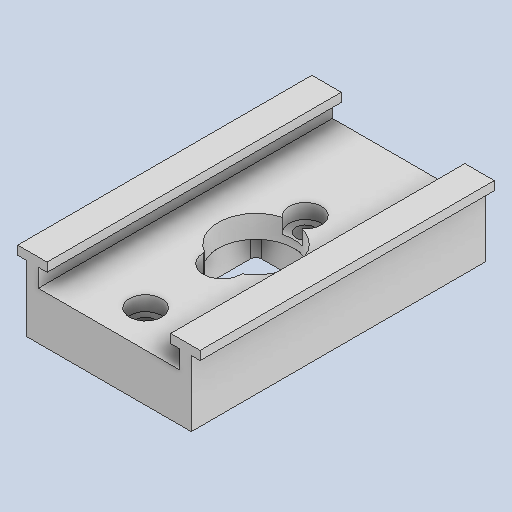
# Autodesk Inventor part: sg90 claw v2
Saved by Autodesk Inventor 2025 (Build 290162000, 162)
## iProperties
Created: 2025-05-11
Part Number: sg90 claw v2
Material: 一般
Document SubType Name: Modeling
Designer: gavin
Density: 1 g/cm^3
Appearance: 預設
Author: gavin
## iProperties of the stored document sg90 claw v2_3D 列印.ipt
Created: 2025-05-11
Part Number: sg90 claw v2_3D 列印
Material: 一般
Document SubType Name: Modeling
Designer: gavin
Density: 1 g/cm^3
Appearance: 預設
Author: gavin
Autodesk Inventor part; units mm, degrees
ref_plane "YZ Plane" through (0, 0, 0) normal (1, 0, 0) x (0, 1, 0)
sketch "草圖1" plane through (0, 0, 0) normal (0, 1, 0) x (-1, 0, 0)
  line L0 (-11.557, 4.8514) -> (-6.731, 4.8514) construction
  arc A0 (-11.557, 4.8514) -> (-12.192, 4.2164) centre (-11.557, 4.2164) ccw construction
  line L1 (-12.192, 4.2164) -> (-12.192, -0.635) construction
  arc A1 (-11.557, 0) -> (-12.192, -0.635) centre (-11.557, -0.635) ccw construction
  line L2 (-11.557, 0) -> (-0.635, 0) construction
  arc A2 (0, -0.635) -> (-0.635, 0) centre (-0.635, -0.635) ccw construction
  line L3 (0, 4.2164) -> (0, -0.635) construction
  arc A3 (0, 4.2164) -> (-0.635, 4.8514) centre (-0.635, 4.2164) ccw construction
  line L4 (-5.461, 4.8514) -> (-0.635, 4.8514) construction
  line L5 (-5.461, 4.0821) -> (-5.461, 4.8514) construction
  arc A4 (-6.731, 4.0821) -> (-5.461, 4.0821) centre (-6.096, 2.286) ccw construction
  line L6 (-6.731, 4.8514) -> (-6.731, 4.0821) construction
  line L7 (-12.192, -26.797) -> (-12.192, -21.9456) construction
  arc A5 (-12.192, -26.797) -> (-11.557, -27.432) centre (-11.557, -26.797) ccw construction
  line L8 (-11.557, -27.432) -> (-6.731, -27.432) construction
  line L9 (-6.731, -27.432) -> (-6.731, -26.6627) construction
  arc A6 (-5.461, -26.6627) -> (-6.731, -26.6627) centre (-6.096, -24.8666) ccw construction
  line L10 (-5.461, -26.6627) -> (-5.461, -27.432) construction
  line L11 (-5.461, -27.432) -> (-0.635, -27.432) construction
  arc A7 (-0.635, -27.432) -> (0, -26.797) centre (-0.635, -26.797) ccw construction
  line L12 (0, -26.797) -> (0, -21.9456) construction
  arc A8 (-0.635, -22.5806) -> (0, -21.9456) centre (-0.635, -21.9456) ccw construction
  line L13 (-11.557, -22.5806) -> (-0.635, -22.5806) construction
  arc A9 (-12.192, -21.9456) -> (-11.557, -22.5806) centre (-11.557, -21.9456) ccw construction
  line L14 (-20.096, 8.5154) -> (7.904, 8.5154)
  line L15 (7.904, 8.5154) -> (7.904, -41.4846)
  line L16 (7.904, -41.4846) -> (-20.096, -41.4846)
  line L17 (-20.096, -41.4846) -> (-20.096, 8.5154)
  line L18 (-20.096, 8.5154) -> (7.904, -41.4846) construction
  line L19 (7.904, 8.5154) -> (-20.096, -41.4846) construction
  arc A10 (-3.2258, -10.7188) -> (-8.9662, -10.7188) centre (-6.096, -10.7188) ccw construction
  line L20 (-8.9662, -10.7188) -> (-8.9662, -11.1066) construction
  arc A11 (-8.9662, -11.1066) -> (-3.2258, -11.1066) centre (-6.096, -16.4846) ccw construction
  line L21 (-3.2258, -11.1066) -> (-3.2258, -10.7188) construction
  arc A12 (-7.0699, -18.6923) -> (-7.0447, -18.7033) centre (-6.096, -16.4846) ccw construction
  spline S0 degree 3 poles (-7.0947, -18.3987) (-7.1625, -18.5159) (-7.1542, -18.6137) (-7.0699, -18.6923) knots 0.499854 0.499854 0.499854 0.499854 0.500096 0.500096 0.500096 0.500096 construction
  arc A13 (-7.336, -18.252) -> (-7.0947, -18.3987) centre (-6.096, -16.4846) ccw construction
  spline S1 degree 3 poles (-7.6081, -18.365) (-7.4996, -18.4037) (-7.4089, -18.3661) (-7.336, -18.252) knots 0.499904 0.499904 0.499904 0.499904 0.500146 0.500146 0.500146 0.500146 construction
  arc A14 (-7.6294, -18.3477) -> (-7.6081, -18.365) centre (-6.096, -16.4846) ccw construction
  spline S2 degree 3 poles (-7.5741, -18.0583) (-7.671, -18.1528) (-7.6894, -18.2493) (-7.6294, -18.3477) knots 0.499854 0.499854 0.499854 0.499854 0.500096 0.500096 0.500096 0.500096 construction
  arc A15 (-7.7669, -17.8519) -> (-7.5741, -18.0583) centre (-6.096, -16.4846) ccw construction
  spline S3 degree 3 poles (-8.0594, -17.8873) (-7.9653, -17.9539) (-7.8678, -17.9421) (-7.7669, -17.8519) knots 0.499904 0.499904 0.499904 0.499904 0.500146 0.500146 0.500146 0.500146 construction
  arc A16 (-8.0752, -17.8649) -> (-8.0594, -17.8873) centre (-6.096, -16.4846) ccw construction
  spline S4 degree 3 poles (-7.9439, -17.6011) (-8.0627, -17.666) (-8.1064, -17.7539) (-8.0752, -17.8649) knots 0.499854 0.499854 0.499854 0.499854 0.500096 0.500096 0.500096 0.500096 construction
  arc A17 (-8.0738, -17.3504) -> (-7.9439, -17.6011) centre (-6.096, -16.4846) ccw construction
  spline S5 degree 3 poles (-8.365, -17.3056) (-8.2924, -17.3951) (-8.1953, -17.41) (-8.0738, -17.3504) knots 0.499904 0.499904 0.499904 0.499904 0.500146 0.500146 0.500146 0.500146 construction
  arc A18 (-8.3742, -17.2797) -> (-8.365, -17.3056) centre (-6.096, -16.4846) ccw construction
  spline S6 degree 3 poles (-8.1766, -17.0612) (-8.3085, -17.0916) (-8.3744, -17.1644) (-8.3742, -17.2797) knots 0.499854 0.499854 0.499854 0.499854 0.500096 0.500096 0.500096 0.500096 construction
  arc A19 (-8.234, -16.7847) -> (-8.1766, -17.0612) centre (-6.096, -16.4846) ccw construction
  spline S7 degree 3 poles (-8.5024, -16.663) (-8.4566, -16.7687) (-8.3671, -16.8093) (-8.234, -16.7847) knots 0.499904 0.499904 0.499904 0.499904 0.500146 0.500146 0.500146 0.500146 construction
  arc A20 (-8.5043, -16.6356) -> (-8.5024, -16.663) centre (-6.096, -16.4846) ccw construction
  spline S8 degree 3 poles (-8.255, -16.4785) (-8.3902, -16.4722) (-8.4733, -16.5245) (-8.5043, -16.6356) knots 0.499854 0.499854 0.499854 0.499854 0.500096 0.500096 0.500096 0.500096 construction
  arc A21 (-8.2357, -16.1967) -> (-8.255, -16.4785) centre (-6.096, -16.4846) ccw construction
  spline S9 degree 3 poles (-8.4613, -16.0071) (-8.4457, -16.1213) (-8.3705, -16.1845) (-8.2357, -16.1967) knots 0.499904 0.499904 0.499904 0.499904 0.500146 0.500146 0.500146 0.500146 construction
  arc A22 (-8.4557, -15.9802) -> (-8.4613, -16.0071) centre (-6.096, -16.4846) ccw construction
  spline S10 degree 3 poles (-8.1733, -15.8962) (-8.3018, -15.8537) (-8.3959, -15.8817) (-8.4557, -15.9802) knots 0.499854 0.499854 0.499854 0.499854 0.500096 0.500096 0.500096 0.500096 construction
  arc A23 (-8.0787, -15.6301) -> (-8.1733, -15.8962) centre (-6.096, -16.4846) ccw construction
  spline S11 degree 3 poles (-8.2448, -15.3867) (-8.2606, -15.5008) (-8.2052, -15.582) (-8.0787, -15.6301) knots 0.499904 0.499904 0.499904 0.499904 0.500146 0.500146 0.500146 0.500146 construction
  arc A24 (-8.2321, -15.3623) -> (-8.2448, -15.3867) centre (-6.096, -16.4846) ccw construction
  spline S12 degree 3 poles (-7.9375, -15.3576) (-8.0497, -15.282) (-8.148, -15.2835) (-8.2321, -15.3623) knots 0.499854 0.499854 0.499854 0.499854 0.500096 0.500096 0.500096 0.500096 construction
  arc A25 (-7.7746, -15.1269) -> (-7.9375, -15.3576) centre (-6.096, -16.4846) ccw construction
  spline S13 degree 3 poles (-7.8689, -14.8477) (-7.9149, -14.9533) (-7.8835, -15.0464) (-7.7746, -15.1269) knots 0.499904 0.499904 0.499904 0.499904 0.500146 0.500146 0.500146 0.500146 construction
  arc A26 (-7.8501, -14.8276) -> (-7.8689, -14.8477) centre (-6.096, -16.4846) ccw construction
  spline S14 degree 3 poles (-7.5651, -14.9025) (-7.6528, -14.7994) (-7.7478, -14.7745) (-7.8501, -14.8276) knots 0.499854 0.499854 0.499854 0.499854 0.500096 0.500096 0.500096 0.500096 construction
  arc A27 (-7.3461, -14.7243) -> (-7.5651, -14.9025) centre (-6.096, -16.4846) ccw construction
  spline S15 degree 3 poles (-7.3615, -14.4301) (-7.4343, -14.5194) (-7.4292, -14.6175) (-7.3461, -14.7243) knots 0.499904 0.499904 0.499904 0.499904 0.500146 0.500146 0.500146 0.500146 construction
  arc A28 (-7.338, -14.4158) -> (-7.3615, -14.4301) centre (-6.096, -16.4846) ccw construction
  spline S16 degree 3 poles (-7.0838, -14.5648) (-7.1404, -14.4419) (-7.2252, -14.3922) (-7.338, -14.4158) knots 0.499854 0.499854 0.499854 0.499854 0.500096 0.500096 0.500096 0.500096 construction
  arc A29 (-6.8248, -14.4523) -> (-7.0838, -14.5648) centre (-6.096, -16.4846) ccw construction
  spline S17 degree 3 poles (-6.7602, -14.1648) (-6.8545, -14.2312) (-6.876, -14.327) (-6.8248, -14.4523) knots 0.499904 0.499904 0.499904 0.499904 0.500146 0.500146 0.500146 0.500146 construction
  arc A30 (-6.7338, -14.1574) -> (-6.7602, -14.1648) centre (-6.096, -16.4846) ccw construction
  spline S18 degree 3 poles (-6.5292, -14.3695) (-6.5506, -14.2359) (-6.6188, -14.1652) (-6.7338, -14.1574) knots 0.499854 0.499854 0.499854 0.499854 0.500096 0.500096 0.500096 0.500096 construction
  arc A31 (-6.2495, -14.3311) -> (-6.5292, -14.3695) centre (-6.096, -16.4846) ccw construction
  spline S19 degree 3 poles (-6.1097, -14.0716) (-6.2184, -14.1101) (-6.265, -14.1966) (-6.2495, -14.3311) knots 0.499904 0.499904 0.499904 0.499904 0.500146 0.500146 0.500146 0.500146 construction
  arc A32 (-6.0823, -14.0716) -> (-6.1097, -14.0716) centre (-6.096, -16.4846) ccw construction
  spline S20 degree 3 poles (-5.9425, -14.3311) (-5.927, -14.1966) (-5.9736, -14.1101) (-6.0823, -14.0716) knots 0.499854 0.499854 0.499854 0.499854 0.500096 0.500096 0.500096 0.500096 construction
  arc A33 (-5.6628, -14.3695) -> (-5.9425, -14.3311) centre (-6.096, -16.4846) ccw construction
  spline S21 degree 3 poles (-5.4582, -14.1574) (-5.5732, -14.1652) (-5.6414, -14.2359) (-5.6628, -14.3695) knots 0.499904 0.499904 0.499904 0.499904 0.500146 0.500146 0.500146 0.500146 construction
  arc A34 (-5.4318, -14.1648) -> (-5.4582, -14.1574) centre (-6.096, -16.4846) ccw construction
  spline S22 degree 3 poles (-5.3672, -14.4523) (-5.316, -14.327) (-5.3375, -14.2312) (-5.4318, -14.1648) knots 0.499854 0.499854 0.499854 0.499854 0.500096 0.500096 0.500096 0.500096 construction
  arc A35 (-5.1082, -14.5648) -> (-5.3672, -14.4523) centre (-6.096, -16.4846) ccw construction
  spline S23 degree 3 poles (-4.854, -14.4158) (-4.9668, -14.3922) (-5.0516, -14.4419) (-5.1082, -14.5648) knots 0.499904 0.499904 0.499904 0.499904 0.500146 0.500146 0.500146 0.500146 construction
  arc A36 (-4.8305, -14.4301) -> (-4.854, -14.4158) centre (-6.096, -16.4846) ccw construction
  spline S24 degree 3 poles (-4.8459, -14.7243) (-4.7628, -14.6175) (-4.7577, -14.5194) (-4.8305, -14.4301) knots 0.499854 0.499854 0.499854 0.499854 0.500096 0.500096 0.500096 0.500096 construction
  arc A37 (-4.6269, -14.9025) -> (-4.8459, -14.7243) centre (-6.096, -16.4846) ccw construction
  spline S25 degree 3 poles (-4.3419, -14.8276) (-4.4442, -14.7745) (-4.5392, -14.7994) (-4.6269, -14.9025) knots 0.499904 0.499904 0.499904 0.499904 0.500146 0.500146 0.500146 0.500146 construction
  arc A38 (-4.3231, -14.8477) -> (-4.3419, -14.8276) centre (-6.096, -16.4846) ccw construction
  spline S26 degree 3 poles (-4.4174, -15.1269) (-4.3085, -15.0464) (-4.2771, -14.9533) (-4.3231, -14.8477) knots 0.499854 0.499854 0.499854 0.499854 0.500096 0.500096 0.500096 0.500096 construction
  arc A39 (-4.2545, -15.3576) -> (-4.4174, -15.1269) centre (-6.096, -16.4846) ccw construction
  spline S27 degree 3 poles (-3.9599, -15.3623) (-4.044, -15.2835) (-4.1423, -15.282) (-4.2545, -15.3576) knots 0.499904 0.499904 0.499904 0.499904 0.500146 0.500146 0.500146 0.500146 construction
  arc A40 (-3.9472, -15.3867) -> (-3.9599, -15.3623) centre (-6.096, -16.4846) ccw construction
  spline S28 degree 3 poles (-4.1133, -15.6301) (-3.9868, -15.582) (-3.9314, -15.5008) (-3.9472, -15.3867) knots 0.499854 0.499854 0.499854 0.499854 0.500096 0.500096 0.500096 0.500096 construction
  arc A41 (-4.0187, -15.8962) -> (-4.1133, -15.6301) centre (-6.096, -16.4846) ccw construction
  spline S29 degree 3 poles (-3.7363, -15.9802) (-3.7961, -15.8817) (-3.8902, -15.8537) (-4.0187, -15.8962) knots 0.499904 0.499904 0.499904 0.499904 0.500146 0.500146 0.500146 0.500146 construction
  arc A42 (-3.7307, -16.0071) -> (-3.7363, -15.9802) centre (-6.096, -16.4846) ccw construction
  spline S30 degree 3 poles (-3.9563, -16.1967) (-3.8215, -16.1845) (-3.7463, -16.1213) (-3.7307, -16.0071) knots 0.499854 0.499854 0.499854 0.499854 0.500096 0.500096 0.500096 0.500096 construction
  arc A43 (-3.937, -16.4785) -> (-3.9563, -16.1967) centre (-6.096, -16.4846) ccw construction
  spline S31 degree 3 poles (-3.6877, -16.6356) (-3.7187, -16.5245) (-3.8018, -16.4722) (-3.937, -16.4785) knots 0.499904 0.499904 0.499904 0.499904 0.500146 0.500146 0.500146 0.500146 construction
  arc A44 (-3.6896, -16.663) -> (-3.6877, -16.6356) centre (-6.096, -16.4846) ccw construction
  spline S32 degree 3 poles (-3.958, -16.7847) (-3.8249, -16.8093) (-3.7354, -16.7687) (-3.6896, -16.663) knots 0.499854 0.499854 0.499854 0.499854 0.500096 0.500096 0.500096 0.500096 construction
  arc A45 (-4.0154, -17.0612) -> (-3.958, -16.7847) centre (-6.096, -16.4846) ccw construction
  spline S33 degree 3 poles (-3.8178, -17.2797) (-3.8176, -17.1644) (-3.8835, -17.0916) (-4.0154, -17.0612) knots 0.499904 0.499904 0.499904 0.499904 0.500146 0.500146 0.500146 0.500146 construction
  arc A46 (-3.827, -17.3056) -> (-3.8178, -17.2797) centre (-6.096, -16.4846) ccw construction
  spline S34 degree 3 poles (-4.1182, -17.3504) (-3.9967, -17.41) (-3.8996, -17.3951) (-3.827, -17.3056) knots 0.499854 0.499854 0.499854 0.499854 0.500096 0.500096 0.500096 0.500096 construction
  arc A47 (-4.2481, -17.6011) -> (-4.1182, -17.3504) centre (-6.096, -16.4846) ccw construction
  spline S35 degree 3 poles (-4.1168, -17.8649) (-4.0856, -17.7539) (-4.1293, -17.666) (-4.2481, -17.6011) knots 0.499904 0.499904 0.499904 0.499904 0.500146 0.500146 0.500146 0.500146 construction
  arc A48 (-4.1326, -17.8873) -> (-4.1168, -17.8649) centre (-6.096, -16.4846) ccw construction
  spline S36 degree 3 poles (-4.4251, -17.8519) (-4.3242, -17.9421) (-4.2267, -17.9539) (-4.1326, -17.8873) knots 0.499854 0.499854 0.499854 0.499854 0.500096 0.500096 0.500096 0.500096 construction
  arc A49 (-4.6179, -18.0583) -> (-4.4251, -17.8519) centre (-6.096, -16.4846) ccw construction
  spline S37 degree 3 poles (-4.5626, -18.3477) (-4.5026, -18.2493) (-4.521, -18.1528) (-4.6179, -18.0583) knots 0.499904 0.499904 0.499904 0.499904 0.500146 0.500146 0.500146 0.500146 construction
  arc A50 (-4.5839, -18.365) -> (-4.5626, -18.3477) centre (-6.096, -16.4846) ccw construction
  spline S38 degree 3 poles (-4.856, -18.252) (-4.7831, -18.3661) (-4.6924, -18.4037) (-4.5839, -18.365) knots 0.499854 0.499854 0.499854 0.499854 0.500096 0.500096 0.500096 0.500096 construction
  arc A51 (-5.0973, -18.3987) -> (-4.856, -18.252) centre (-6.096, -16.4846) ccw construction
  spline S39 degree 3 poles (-5.1221, -18.6923) (-5.0378, -18.6137) (-5.0295, -18.5159) (-5.0973, -18.3987) knots 0.499904 0.499904 0.499904 0.499904 0.500146 0.500146 0.500146 0.500146 construction
  arc A52 (-5.1473, -18.7033) -> (-5.1221, -18.6923) centre (-6.096, -16.4846) ccw construction
  spline S40 degree 3 poles (-5.3788, -18.521) (-5.3394, -18.6505) (-5.2623, -18.7113) (-5.1473, -18.7033) knots 0.499854 0.499854 0.499854 0.499854 0.500096 0.500096 0.500096 0.500096 construction
  arc A53 (-5.6507, -18.5972) -> (-5.3788, -18.521) centre (-6.096, -16.4846) ccw construction
  spline S41 degree 3 poles (-5.7538, -18.8732) (-5.6514, -18.8203) (-5.6171, -18.7283) (-5.6507, -18.5972) knots 0.499904 0.499904 0.499904 0.499904 0.500146 0.500146 0.500146 0.500146 construction
  arc A54 (-5.781, -18.877) -> (-5.7538, -18.8732) centre (-6.096, -16.4846) ccw construction
  spline S42 degree 3 poles (-5.9548, -18.639) (-5.9518, -18.7743) (-5.8939, -18.8536) (-5.781, -18.877) knots 0.499854 0.499854 0.499854 0.499854 0.500096 0.500096 0.500096 0.500096 construction
  arc A55 (-6.2372, -18.639) -> (-5.9548, -18.639) centre (-6.096, -16.4846) ccw construction
  spline S43 degree 3 poles (-6.411, -18.877) (-6.2981, -18.8536) (-6.2402, -18.7743) (-6.2372, -18.639) knots 0.499904 0.499904 0.499904 0.499904 0.500146 0.500146 0.500146 0.500146 construction
  arc A56 (-6.4382, -18.8732) -> (-6.411, -18.877) centre (-6.096, -16.4846) ccw construction
  spline S44 degree 3 poles (-6.5413, -18.5972) (-6.5749, -18.7283) (-6.5406, -18.8203) (-6.4382, -18.8732) knots 0.499854 0.499854 0.499854 0.499854 0.500096 0.500096 0.500096 0.500096 construction
  arc A57 (-6.8132, -18.521) -> (-6.5413, -18.5972) centre (-6.096, -16.4846) ccw construction
  spline S45 degree 3 poles (-7.0447, -18.7033) (-6.9297, -18.7113) (-6.8526, -18.6505) (-6.8132, -18.521) knots 0.499904 0.499904 0.499904 0.499904 0.500146 0.500146 0.500146 0.500146 construction
  line L22 (0, -16.4846) -> (0, -0.635) construction
  arc A58 (0, -0.635) -> (-0.635, 0) centre (-0.635, -0.635) ccw construction
  line L23 (-0.635, 0) -> (-11.557, 0) construction
  arc A59 (-11.557, 0) -> (-12.192, -0.635) centre (-11.557, -0.635) ccw construction
  line L24 (-12.192, -0.635) -> (-12.192, -16.4846) construction
  arc A60 (-8.9662, -11.1066) -> (-12.192, -16.4846) centre (-6.096, -16.4846) ccw construction
  line L25 (-8.9662, -10.7188) -> (-8.9662, -11.1066) construction
  arc A61 (-3.2258, -10.7188) -> (-8.9662, -10.7188) centre (-6.096, -10.7188) ccw construction
  line L26 (-3.2258, -11.1066) -> (-3.2258, -10.7188) construction
  arc A62 (0, -16.4846) -> (-3.2258, -11.1066) centre (-6.096, -16.4846) ccw construction
  line L27 (-6.096, -22.5806) -> (-0.635, -22.5806) construction
  arc A63 (-0.635, -22.5806) -> (0, -21.9456) centre (-0.635, -21.9456) ccw construction
  line L28 (0, -21.9456) -> (0, -16.4846) construction
  arc A64 (-6.096, -22.5806) -> (0, -16.4846) centre (-6.096, -16.4846) ccw construction
  line L29 (-12.192, -16.4846) -> (-12.192, -21.9456) construction
  arc A65 (-12.192, -21.9456) -> (-11.557, -22.5806) centre (-11.557, -21.9456) ccw construction
  line L30 (-11.557, -22.5806) -> (-6.096, -22.5806) construction
  arc A66 (-12.192, -16.4846) -> (-6.096, -22.5806) centre (-6.096, -16.4846) ccw construction
  line L31 (0.3, -0.635) -> (0.3, -16.4846)
  line L32 (0.3, -16.4846) -> (0.3, -21.9456)
  arc A67 (-0.635, -22.8806) -> (0.3, -21.9456) centre (-0.635, -21.9456) ccw
  line L33 (-0.635, -22.8806) -> (-6.096, -22.8806)
  line L34 (-6.096, -22.8806) -> (-11.557, -22.8806)
  arc A68 (-12.492, -21.9456) -> (-11.557, -22.8806) centre (-11.557, -21.9456) ccw
  line L35 (-12.492, -21.9456) -> (-12.492, -16.4846)
  line L36 (-12.492, -16.4846) -> (-12.492, -0.635)
  arc A69 (-11.557, 0.3) -> (-12.492, -0.635) centre (-11.557, -0.635) ccw
  line L37 (-11.557, 0.3) -> (-0.635, 0.3)
  arc A70 (0.3, -0.635) -> (-0.635, 0.3) centre (-0.635, -0.635) ccw
  circle A71 centre (-6.096, 2.286) radius 1.6
  circle A72 centre (-6.096, -24.8666) radius 1.6
  point P0 (0, 0)
  dimension "d0" = 28
  dimension "d1" = 50
  dimension "d2" = 0.3
  dimension "d3" = 3.2
  dimension "d4" = 3.2
  constraints: 26 end point, 8 point on circle, 6 centre point, 3 coincident, 2 midpoint, 2 parallel, 1 horizontal, 1 perpendicular, 10 other
  measures "d0" distance of L15.end L16.end
  measures "d1" distance of L14.end L15.end
  measures "d2" distance between parallel lines of L22 L31
  measures "d3" diameter of A71
  measures "d4" diameter of A72
ref_plane "工作平面1" through (0, -4.2926, -0.635) normal (0, 1, 0) x (0, 0, 1)
extrude "擠出1" add sketch "草圖1" against normal up to surface (4.2926 mm away)
sketch "草圖2" plane through (0, 0, 0) normal (0, 1, 0) x (1, 0, 0)
  line L0 (20.096, 41.4846) -> (-7.904, 41.4846) projected
  line L1 (-7.904, 41.4846) -> (-7.904, -8.5154) projected
  line L2 (-7.904, -8.5154) -> (20.096, -8.5154) projected
  line L3 (20.096, -8.5154) -> (20.096, 41.4846) projected
  line L4 (11.557, -0.3) -> (0.635, -0.3) construction
  arc A0 (-0.3, 0.635) -> (0.635, -0.3) centre (0.635, 0.635) ccw construction
  line L5 (-0.3, 0.635) -> (-0.3, 21.9456) construction
  arc A1 (0.635, 22.8806) -> (-0.3, 21.9456) centre (0.635, 21.9456) ccw construction
  line L6 (0.635, 22.8806) -> (11.557, 22.8806) construction
  arc A2 (12.492, 21.9456) -> (11.557, 22.8806) centre (11.557, 21.9456) ccw construction
  line L7 (12.492, 21.9456) -> (12.492, 0.635) construction
  arc A3 (11.557, -0.3) -> (12.492, 0.635) centre (11.557, 0.635) ccw construction
  circle A4 centre (6.096, 24.8666) radius 1.6 projected
  circle A5 centre (6.096, -2.286) radius 1.6 projected
  arc A6 (3.2258, 10.7188) -> (8.9662, 10.7188) centre (6.096, 10.7188) ccw projected
  line L8 (8.9662, 10.7188) -> (8.9662, 11.1066) projected
  arc A7 (8.9662, 11.1066) -> (3.2258, 11.1066) centre (6.096, 16.4846) ccw projected
  line L9 (3.2258, 11.1066) -> (3.2258, 10.7188) projected
  arc A8 (7.0699, 18.6923) -> (7.0447, 18.7033) centre (6.096, 16.4846) ccw projected
  spline S0 degree 3 poles (7.0947, 18.3987) (7.1625, 18.5159) (7.1542, 18.6137) (7.0699, 18.6923) knots 0.499854 0.499854 0.499854 0.499854 0.500096 0.500096 0.500096 0.500096 projected
  arc A9 (7.336, 18.252) -> (7.0947, 18.3987) centre (6.096, 16.4846) ccw projected
  spline S1 degree 3 poles (7.6081, 18.365) (7.4996, 18.4037) (7.4089, 18.3661) (7.336, 18.252) knots 0.499904 0.499904 0.499904 0.499904 0.500146 0.500146 0.500146 0.500146 projected
  arc A10 (7.6294, 18.3477) -> (7.6081, 18.365) centre (6.096, 16.4846) ccw projected
  spline S2 degree 3 poles (7.5741, 18.0583) (7.671, 18.1528) (7.6894, 18.2493) (7.6294, 18.3477) knots 0.499854 0.499854 0.499854 0.499854 0.500096 0.500096 0.500096 0.500096 projected
  arc A11 (7.7669, 17.8519) -> (7.5741, 18.0583) centre (6.096, 16.4846) ccw projected
  spline S3 degree 3 poles (8.0594, 17.8873) (7.9653, 17.9539) (7.8678, 17.9421) (7.7669, 17.8519) knots 0.499904 0.499904 0.499904 0.499904 0.500146 0.500146 0.500146 0.500146 projected
  arc A12 (8.0752, 17.8649) -> (8.0594, 17.8873) centre (6.096, 16.4846) ccw projected
  spline S4 degree 3 poles (7.9439, 17.6011) (8.0627, 17.666) (8.1064, 17.7539) (8.0752, 17.8649) knots 0.499854 0.499854 0.499854 0.499854 0.500096 0.500096 0.500096 0.500096 projected
  arc A13 (8.0738, 17.3504) -> (7.9439, 17.6011) centre (6.096, 16.4846) ccw projected
  spline S5 degree 3 poles (8.365, 17.3056) (8.2924, 17.3951) (8.1953, 17.41) (8.0738, 17.3504) knots 0.499904 0.499904 0.499904 0.499904 0.500146 0.500146 0.500146 0.500146 projected
  arc A14 (8.3742, 17.2797) -> (8.365, 17.3056) centre (6.096, 16.4846) ccw projected
  spline S6 degree 3 poles (8.1766, 17.0612) (8.3085, 17.0916) (8.3744, 17.1644) (8.3742, 17.2797) knots 0.499854 0.499854 0.499854 0.499854 0.500096 0.500096 0.500096 0.500096 projected
  arc A15 (8.234, 16.7847) -> (8.1766, 17.0612) centre (6.096, 16.4846) ccw projected
  spline S7 degree 3 poles (8.5024, 16.663) (8.4566, 16.7687) (8.3671, 16.8093) (8.234, 16.7847) knots 0.499904 0.499904 0.499904 0.499904 0.500146 0.500146 0.500146 0.500146 projected
  arc A16 (8.5043, 16.6356) -> (8.5024, 16.663) centre (6.096, 16.4846) ccw projected
  spline S8 degree 3 poles (8.255, 16.4785) (8.3902, 16.4722) (8.4733, 16.5245) (8.5043, 16.6356) knots 0.499854 0.499854 0.499854 0.499854 0.500096 0.500096 0.500096 0.500096 projected
  arc A17 (8.2357, 16.1967) -> (8.255, 16.4785) centre (6.096, 16.4846) ccw projected
  spline S9 degree 3 poles (8.4613, 16.0071) (8.4457, 16.1213) (8.3705, 16.1845) (8.2357, 16.1967) knots 0.499904 0.499904 0.499904 0.499904 0.500146 0.500146 0.500146 0.500146 projected
  arc A18 (8.4557, 15.9802) -> (8.4613, 16.0071) centre (6.096, 16.4846) ccw projected
  spline S10 degree 3 poles (8.1733, 15.8962) (8.3018, 15.8537) (8.3959, 15.8817) (8.4557, 15.9802) knots 0.499854 0.499854 0.499854 0.499854 0.500096 0.500096 0.500096 0.500096 projected
  arc A19 (8.0787, 15.6301) -> (8.1733, 15.8962) centre (6.096, 16.4846) ccw projected
  spline S11 degree 3 poles (8.2448, 15.3867) (8.2606, 15.5008) (8.2052, 15.582) (8.0787, 15.6301) knots 0.499904 0.499904 0.499904 0.499904 0.500146 0.500146 0.500146 0.500146 projected
  arc A20 (8.2321, 15.3623) -> (8.2448, 15.3867) centre (6.096, 16.4846) ccw projected
  spline S12 degree 3 poles (7.9375, 15.3576) (8.0497, 15.282) (8.148, 15.2835) (8.2321, 15.3623) knots 0.499854 0.499854 0.499854 0.499854 0.500096 0.500096 0.500096 0.500096 projected
  arc A21 (7.7746, 15.1269) -> (7.9375, 15.3576) centre (6.096, 16.4846) ccw projected
  spline S13 degree 3 poles (7.8689, 14.8477) (7.9149, 14.9533) (7.8835, 15.0464) (7.7746, 15.1269) knots 0.499904 0.499904 0.499904 0.499904 0.500146 0.500146 0.500146 0.500146 projected
  arc A22 (7.8501, 14.8276) -> (7.8689, 14.8477) centre (6.096, 16.4846) ccw projected
  spline S14 degree 3 poles (7.5651, 14.9025) (7.6528, 14.7994) (7.7478, 14.7745) (7.8501, 14.8276) knots 0.499854 0.499854 0.499854 0.499854 0.500096 0.500096 0.500096 0.500096 projected
  arc A23 (7.3461, 14.7243) -> (7.5651, 14.9025) centre (6.096, 16.4846) ccw projected
  spline S15 degree 3 poles (7.3615, 14.4301) (7.4343, 14.5194) (7.4292, 14.6175) (7.3461, 14.7243) knots 0.499904 0.499904 0.499904 0.499904 0.500146 0.500146 0.500146 0.500146 projected
  arc A24 (7.338, 14.4158) -> (7.3615, 14.4301) centre (6.096, 16.4846) ccw projected
  spline S16 degree 3 poles (7.0838, 14.5648) (7.1404, 14.4419) (7.2252, 14.3922) (7.338, 14.4158) knots 0.499854 0.499854 0.499854 0.499854 0.500096 0.500096 0.500096 0.500096 projected
  arc A25 (6.8248, 14.4523) -> (7.0838, 14.5648) centre (6.096, 16.4846) ccw projected
  spline S17 degree 3 poles (6.7602, 14.1648) (6.8545, 14.2312) (6.876, 14.327) (6.8248, 14.4523) knots 0.499904 0.499904 0.499904 0.499904 0.500146 0.500146 0.500146 0.500146 projected
  arc A26 (6.7338, 14.1574) -> (6.7602, 14.1648) centre (6.096, 16.4846) ccw projected
  spline S18 degree 3 poles (6.5292, 14.3695) (6.5506, 14.2359) (6.6188, 14.1652) (6.7338, 14.1574) knots 0.499854 0.499854 0.499854 0.499854 0.500096 0.500096 0.500096 0.500096 projected
  arc A27 (6.2495, 14.3311) -> (6.5292, 14.3695) centre (6.096, 16.4846) ccw projected
  spline S19 degree 3 poles (6.1097, 14.0716) (6.2184, 14.1101) (6.265, 14.1966) (6.2495, 14.3311) knots 0.499904 0.499904 0.499904 0.499904 0.500146 0.500146 0.500146 0.500146 projected
  arc A28 (6.0823, 14.0716) -> (6.1097, 14.0716) centre (6.096, 16.4846) ccw projected
  spline S20 degree 3 poles (5.9425, 14.3311) (5.927, 14.1966) (5.9736, 14.1101) (6.0823, 14.0716) knots 0.499854 0.499854 0.499854 0.499854 0.500096 0.500096 0.500096 0.500096 projected
  arc A29 (5.6628, 14.3695) -> (5.9425, 14.3311) centre (6.096, 16.4846) ccw projected
  spline S21 degree 3 poles (5.4582, 14.1574) (5.5732, 14.1652) (5.6414, 14.2359) (5.6628, 14.3695) knots 0.499904 0.499904 0.499904 0.499904 0.500146 0.500146 0.500146 0.500146 projected
  arc A30 (5.4318, 14.1648) -> (5.4582, 14.1574) centre (6.096, 16.4846) ccw projected
  spline S22 degree 3 poles (5.3672, 14.4523) (5.316, 14.327) (5.3375, 14.2312) (5.4318, 14.1648) knots 0.499854 0.499854 0.499854 0.499854 0.500096 0.500096 0.500096 0.500096 projected
  arc A31 (5.1082, 14.5648) -> (5.3672, 14.4523) centre (6.096, 16.4846) ccw projected
  spline S23 degree 3 poles (4.854, 14.4158) (4.9668, 14.3922) (5.0516, 14.4419) (5.1082, 14.5648) knots 0.499904 0.499904 0.499904 0.499904 0.500146 0.500146 0.500146 0.500146 projected
  arc A32 (4.8305, 14.4301) -> (4.854, 14.4158) centre (6.096, 16.4846) ccw projected
  spline S24 degree 3 poles (4.8459, 14.7243) (4.7628, 14.6175) (4.7577, 14.5194) (4.8305, 14.4301) knots 0.499854 0.499854 0.499854 0.499854 0.500096 0.500096 0.500096 0.500096 projected
  arc A33 (4.6269, 14.9025) -> (4.8459, 14.7243) centre (6.096, 16.4846) ccw projected
  spline S25 degree 3 poles (4.3419, 14.8276) (4.4442, 14.7745) (4.5392, 14.7994) (4.6269, 14.9025) knots 0.499904 0.499904 0.499904 0.499904 0.500146 0.500146 0.500146 0.500146 projected
  arc A34 (4.3231, 14.8477) -> (4.3419, 14.8276) centre (6.096, 16.4846) ccw projected
  spline S26 degree 3 poles (4.4174, 15.1269) (4.3085, 15.0464) (4.2771, 14.9533) (4.3231, 14.8477) knots 0.499854 0.499854 0.499854 0.499854 0.500096 0.500096 0.500096 0.500096 projected
  arc A35 (4.2545, 15.3576) -> (4.4174, 15.1269) centre (6.096, 16.4846) ccw projected
  spline S27 degree 3 poles (3.9599, 15.3623) (4.044, 15.2835) (4.1423, 15.282) (4.2545, 15.3576) knots 0.499904 0.499904 0.499904 0.499904 0.500146 0.500146 0.500146 0.500146 projected
  arc A36 (3.9472, 15.3867) -> (3.9599, 15.3623) centre (6.096, 16.4846) ccw projected
  spline S28 degree 3 poles (4.1133, 15.6301) (3.9868, 15.582) (3.9314, 15.5008) (3.9472, 15.3867) knots 0.499854 0.499854 0.499854 0.499854 0.500096 0.500096 0.500096 0.500096 projected
  arc A37 (4.0187, 15.8962) -> (4.1133, 15.6301) centre (6.096, 16.4846) ccw projected
  spline S29 degree 3 poles (3.7363, 15.9802) (3.7961, 15.8817) (3.8902, 15.8537) (4.0187, 15.8962) knots 0.499904 0.499904 0.499904 0.499904 0.500146 0.500146 0.500146 0.500146 projected
  arc A38 (3.7307, 16.0071) -> (3.7363, 15.9802) centre (6.096, 16.4846) ccw projected
  spline S30 degree 3 poles (3.9563, 16.1967) (3.8215, 16.1845) (3.7463, 16.1213) (3.7307, 16.0071) knots 0.499854 0.499854 0.499854 0.499854 0.500096 0.500096 0.500096 0.500096 projected
  arc A39 (3.937, 16.4785) -> (3.9563, 16.1967) centre (6.096, 16.4846) ccw projected
  spline S31 degree 3 poles (3.6877, 16.6356) (3.7187, 16.5245) (3.8018, 16.4722) (3.937, 16.4785) knots 0.499904 0.499904 0.499904 0.499904 0.500146 0.500146 0.500146 0.500146 projected
  arc A40 (3.6896, 16.663) -> (3.6877, 16.6356) centre (6.096, 16.4846) ccw projected
  spline S32 degree 3 poles (3.958, 16.7847) (3.8249, 16.8093) (3.7354, 16.7687) (3.6896, 16.663) knots 0.499854 0.499854 0.499854 0.499854 0.500096 0.500096 0.500096 0.500096 projected
  arc A41 (4.0154, 17.0612) -> (3.958, 16.7847) centre (6.096, 16.4846) ccw projected
  spline S33 degree 3 poles (3.8178, 17.2797) (3.8176, 17.1644) (3.8835, 17.0916) (4.0154, 17.0612) knots 0.499904 0.499904 0.499904 0.499904 0.500146 0.500146 0.500146 0.500146 projected
  arc A42 (3.827, 17.3056) -> (3.8178, 17.2797) centre (6.096, 16.4846) ccw projected
  spline S34 degree 3 poles (4.1182, 17.3504) (3.9967, 17.41) (3.8996, 17.3951) (3.827, 17.3056) knots 0.499854 0.499854 0.499854 0.499854 0.500096 0.500096 0.500096 0.500096 projected
  arc A43 (4.2481, 17.6011) -> (4.1182, 17.3504) centre (6.096, 16.4846) ccw projected
  spline S35 degree 3 poles (4.1168, 17.8649) (4.0856, 17.7539) (4.1293, 17.666) (4.2481, 17.6011) knots 0.499904 0.499904 0.499904 0.499904 0.500146 0.500146 0.500146 0.500146 projected
  arc A44 (4.1326, 17.8873) -> (4.1168, 17.8649) centre (6.096, 16.4846) ccw projected
  spline S36 degree 3 poles (4.4251, 17.8519) (4.3242, 17.9421) (4.2267, 17.9539) (4.1326, 17.8873) knots 0.499854 0.499854 0.499854 0.499854 0.500096 0.500096 0.500096 0.500096 projected
  arc A45 (4.6179, 18.0583) -> (4.4251, 17.8519) centre (6.096, 16.4846) ccw projected
  spline S37 degree 3 poles (4.5626, 18.3477) (4.5026, 18.2493) (4.521, 18.1528) (4.6179, 18.0583) knots 0.499904 0.499904 0.499904 0.499904 0.500146 0.500146 0.500146 0.500146 projected
  arc A46 (4.5839, 18.365) -> (4.5626, 18.3477) centre (6.096, 16.4846) ccw projected
  spline S38 degree 3 poles (4.856, 18.252) (4.7831, 18.3661) (4.6924, 18.4037) (4.5839, 18.365) knots 0.499854 0.499854 0.499854 0.499854 0.500096 0.500096 0.500096 0.500096 projected
  arc A47 (5.0973, 18.3987) -> (4.856, 18.252) centre (6.096, 16.4846) ccw projected
  spline S39 degree 3 poles (5.1221, 18.6923) (5.0378, 18.6137) (5.0295, 18.5159) (5.0973, 18.3987) knots 0.499904 0.499904 0.499904 0.499904 0.500146 0.500146 0.500146 0.500146 projected
  arc A48 (5.1473, 18.7033) -> (5.1221, 18.6923) centre (6.096, 16.4846) ccw projected
  spline S40 degree 3 poles (5.3788, 18.521) (5.3394, 18.6505) (5.2623, 18.7113) (5.1473, 18.7033) knots 0.499854 0.499854 0.499854 0.499854 0.500096 0.500096 0.500096 0.500096 projected
  arc A49 (5.6507, 18.5972) -> (5.3788, 18.521) centre (6.096, 16.4846) ccw projected
  spline S41 degree 3 poles (5.7538, 18.8732) (5.6514, 18.8203) (5.6171, 18.7283) (5.6507, 18.5972) knots 0.499904 0.499904 0.499904 0.499904 0.500146 0.500146 0.500146 0.500146 projected
  arc A50 (5.781, 18.877) -> (5.7538, 18.8732) centre (6.096, 16.4846) ccw projected
  spline S42 degree 3 poles (5.9548, 18.639) (5.9518, 18.7743) (5.8939, 18.8536) (5.781, 18.877) knots 0.499854 0.499854 0.499854 0.499854 0.500096 0.500096 0.500096 0.500096 projected
  arc A51 (6.2372, 18.639) -> (5.9548, 18.639) centre (6.096, 16.4846) ccw projected
  spline S43 degree 3 poles (6.411, 18.877) (6.2981, 18.8536) (6.2402, 18.7743) (6.2372, 18.639) knots 0.499904 0.499904 0.499904 0.499904 0.500146 0.500146 0.500146 0.500146 projected
  arc A52 (6.4382, 18.8732) -> (6.411, 18.877) centre (6.096, 16.4846) ccw projected
  spline S44 degree 3 poles (6.5413, 18.5972) (6.5749, 18.7283) (6.5406, 18.8203) (6.4382, 18.8732) knots 0.499854 0.499854 0.499854 0.499854 0.500096 0.500096 0.500096 0.500096 projected
  arc A53 (6.8132, 18.521) -> (6.5413, 18.5972) centre (6.096, 16.4846) ccw projected
  spline S45 degree 3 poles (7.0447, 18.7033) (6.9297, 18.7113) (6.8526, 18.6505) (6.8132, 18.521) knots 0.499904 0.499904 0.499904 0.499904 0.500146 0.500146 0.500146 0.500146 projected
  arc A54 (9.2662, 10.9295) -> (2.9258, 10.9295) centre (6.096, 16.4846) ccw
  line L10 (9.2662, 10.9295) -> (9.2662, 10.7188)
  arc A55 (2.9258, 10.7188) -> (9.2662, 10.7188) centre (6.096, 10.7188) ccw
  line L11 (2.9258, 10.7188) -> (2.9258, 10.9295)
  point P0 (0, 0)
  dimension "d7" = 0.3
  constraints: 4 end point, 4 point on circle, 2 centre point, 3 other
  measures "d7" radial gap between concentric circles of A7 A54
ref_plane "工作平面2" through (0, 3.81, -22.5806) normal (0, 1, 0) x (0, 0, 1)
extrude "擠出2" add sketch "草圖2" along normal up to surface (3.81 mm away) contours L3 L2 L1 L0
sketch "草圖3" plane through (-7.904, 3.81, -41.4846) normal (0, 1, 0) x (1, 0, 0)
  circle A0 centre (14, -43.7706) radius 1.6 projected
  circle A1 centre (14, -16.618) radius 1.6 projected
  circle A2 centre (14, -43.7706) radius 2.75
  circle A3 centre (14, -16.618) radius 2.75
  point P0 (7.904, -41.4846)
  dimension "d10" = 5.5
  dimension "d11" = 5.5
  constraints: 2 centre point, 2 coincident
  measures "d10" diameter of A2
  measures "d11" diameter of A3
extrude "擠出3" cut sketch "草圖3" against normal blind 2.5 contours A0 | A1 | A2 | A3
sketch "草圖4" plane through (-7.904, -4.2926, 8.5154) normal (0, 0, 1) x (1, 0, 0)
  line L0 (28, 8.1026) -> (0, 8.1026) projected
  line L1 (0, 8.1026) -> (0, 11.2055)
  line L2 (0, 11.2055) -> (-1.5, 11.2055)
  line L3 (-1.5, 11.2055) -> (-1.5, 12.7055)
  line L4 (-1.5, 12.7055) -> (3.5, 12.7055)
  line L5 (3.5, 12.7055) -> (3.5, 11.2055)
  line L6 (3.5, 11.2055) -> (2, 11.2055)
  line L7 (2, 11.2055) -> (2, 8.1026)
  line L8 (0, 0) -> (0, 8.1026) projected
  line L9 (14, 8.1026) -> (14, 0)
  line L10 (0, 0) -> (28, 0) projected
  line L11 (28, 8.1026) -> (28, 11.2055)
  line L12 (28, 11.2055) -> (29.5, 11.2055)
  line L13 (29.5, 11.2055) -> (29.5, 12.7055)
  line L14 (29.5, 12.7055) -> (24.5, 12.7055)
  line L15 (24.5, 12.7055) -> (24.5, 11.2055)
  line L16 (24.5, 11.2055) -> (26, 11.2055)
  line L17 (26, 11.2055) -> (26, 8.1026)
  point P0 (7.904, 4.2926)
  point P1 (-0.75, 11.2055)
  point P2 (2.75, 11.2055)
  point P3 (28.75, 11.2055)
  point P4 (25.25, 11.2055)
  point P5 (26, 8.1026)
  point P6 (1, 12.7055)
  dimension "d18" = 2
  dimension "d19" = 1.5
  dimension "d20" = 1.5
  dimension "d21" = 1.5
  dimension "d22" = 1.5
  constraints: 30 end point, 10 symmetric about line, 5 midpoint, 3 perpendicular, 3 point on line, 2 vertical, 1 collinear, 1 horizontal, 1 horizontal alignment
  measures "d18" distance between parallel lines of L7 L1
  measures "d19" distance of L2.end L3.end
  measures "d20" distance of L4.end L5.end
  measures "d21" distance of L1.end L2.end
  measures "d22" distance of L5.end L6.end
extrude "擠出4" add sketch "草圖4" against normal up to surface (50 mm away) contours L0 L17 L16 L15 L14 L13 L12 L11 | L0 L1 L2 L3 L4 L5 L6 L7
